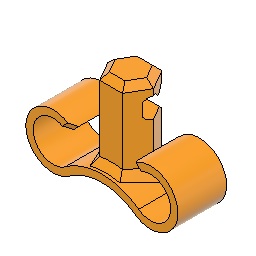
Prusament Clip v6 (Autodesk Fusion 360 design; units mm, degrees)
Autodesk Fusion 360 part; units mm, degrees
note: some values were not read from the file. Chosen so that the rebuilt part matches the saved one: which face or edge a step refers to; which pieces of a blend or face edit are solid. Set by a fixed rule: which sketch regions a step uses.
sketch "Sketch1" plane through (0, 0, 0) normal (0, 0, 1) x (1, 0, 0)
  line L0 (0, 0) -> (-8, 0)
  arc A0 (-5.3, 4.3077) -> (-8, 0) centre (-8, 3) ccw
  arc A1 (-4.22, 4.8307) -> (-8, -1.2) centre (-8, 3) ccw
  line L1 (0, -1.2) -> (-8, -1.2)
  line L2 (-5.3, 4.3077) -> (-4.22, 4.8307)
  line L3 (0, 2.5) -> (0, 20)
  arc A2 (8, 0) -> (5.3, 4.3077) centre (8, 3) ccw
  arc A3 (8, -1.2) -> (4.22, 4.8307) centre (8, 3) ccw
  line L4 (0, 0) -> (8, 0)
  line L5 (0, -1.2) -> (8, -1.2)
  line L6 (5.3, 4.3077) -> (4.22, 4.8307)
  dimension "d1" = 8
  dimension "d2" = 3
  dimension "d3" = 5.3
  dimension "d4" = 1.2
  constraint coincident L0.start L4.start
  constraint horizontal L0
  constraint tangent L0 A0
  constraint symmetric L0.start L3 L4.start
  constraint symmetric L0.end L3 A2.start
  constraint symmetric A0.start L3 A2.end
  constraint symmetric A0 L3 A2
  constraint symmetric A1.end L3 A3.start
  constraint symmetric A1.start L3 A3.end
  constraint symmetric A1 L3 A3
  constraint symmetric L1.start L3 L5.start
  measures "d1" distance of L0.start L0.end
  measures "d2" radius of A0
  measures "d3" horizontal distance of L0.start A0.start
extrude "Extrude1" add sketch "Sketch1" along normal blind 8 makes body 1
sketch "Sketch2" plane through (0, 0, 0) normal (0, 1, 0) x (-1, 0, 0)
  line L0 (-8, 0) -> (8, 0)
  line L1 (8, 0) -> (8, 8)
  line L2 (8, 8) -> (-8, 8)
  line L3 (-8, 8) -> (-8, 0)
  line L4 (1.875, 8) -> (-1.875, 8)
  line L5 (-1.875, 8) -> (-3.75, 4.7524)
  line L6 (-3.75, 4.7524) -> (-1.875, 1.5048)
  line L7 (-1.875, 1.5048) -> (1.875, 1.5048)
  line L8 (1.875, 1.5048) -> (3.75, 4.7524)
  line L9 (3.75, 4.7524) -> (1.875, 8)
  point P0 (0, 4.7524)
  dimension "d12" = 3.75
  constraint collinear L2 L4
  constraint vertical P0 origin
  measures "d12" distance of L4.start P0
extrude "Extrude2" add sketch "Sketch2" along normal blind 16 contours L2 L4 L5 L6 L7 L8 L9 bodies 1
sketch "Sketch5" plane through (0, 0, 1.5048) normal (0, 0, -1) x (-1, 0, 0)
  line L0 (-1.875, 0) -> (1.875, 0)
  line L1 (1.875, 0) -> (1.875, 16)
  line L2 (1.875, 16) -> (-1.875, 16)
  line L3 (-1.875, 16) -> (-1.875, 0)
  line L4 (-3.75, 11.97) -> (-1, 11.97)
  line L5 (-1, 11.97) -> (-1, 12.47)
  arc A0 (1, 12.47) -> (-1, 12.47) centre (0, 12.47) ccw
  line L6 (1, 12.47) -> (1, 9.97)
  line L7 (1, 9.97) -> (-3.75, 9.97)
  line L8 (-3.75, 9.97) -> (-3.75, 11.97)
  line L9 (0, 2.5) -> (0, 20)
  line L10 (-3.75, 0) -> (-3.75, 16) construction
  line L11 (3.75, 0) -> (3.75, 16) construction
  line L12 (0, 0) -> (-8, 0) construction
  point P0 (-3.75, 11.97)
  point P1 (0, 2.5)
  dimension "d27" = 2
  dimension "d29" = 1
  dimension "d30" = 11.97
  dimension "d31" = 0.5
  constraint perpendicular L3 L4
  constraint perpendicular L4 L5
  constraint tangent L5 A0
  constraint perpendicular L5 L7
  constraint parallel L6 L8
  constraint parallel L5 L6
  constraint tangent A0 L6
  constraint vertical A0.centre P1
  constraint coincident P0 L4.start
  constraint collinear L8 L10
  measures "d27" distance of P0 L7.end
  measures "d29" radius of A0
  measures "d30" distance of P0 L12
  measures "d31" distance of L4.end L5.end
extrude "Extrude4" cut sketch "Sketch5" against normal through all contours L3 L4 L7 L8 | L3 L4 L5 A0 L7 L9 | A0 L6 L7 L9 bodies 1
chamfer "Chamfer5" distance 1 angle 45 6 edges at (0, 16, 8) (2.8125, 16, 6.3762) (2.8125, 16, 3.1286) (0, 16, 1.5048) (-2.8125, 16, 3.1286) (-2.8125, 16, 6.3762) on bodies 1
chamfer "Chamfer6" distance 1 angle 45 4 edges at (2.8125, 11.97, 3.1286) (2.8125, 11.97, 6.3762) (2.8125, 9.97, 6.3762) (2.8125, 9.97, 3.1286) on bodies 1
chamfer "Chamfer2" distance 1 angle 45 4 edges at (4.76, 4.5692, 0) (4.76, 4.5692, 8) (-4.76, 4.5692, 8) (-4.76, 4.5692, 0) on bodies 1
fillet "Fillet1" radius 0.8 1 edges at (-1, 9.97, 4.7524) on bodies 1
fillet "Fillet2" radius 3 5 edges at (2.8125, 0, 6.3762) (2.8125, 0, 3.1286) (0, 0, 1.5048) (-2.8125, 0, 3.1286) (-2.8125, 0, 6.3762) on bodies 1
sketch "Sketch1 (2)" plane through (0, 0, 0) normal (0, 0, 1) x (1, 0, 0) in component "Prusa Clip 2"
  circle A0 centre (-8, 0) radius 4.5
  circle A1 centre (8, 0) radius 4.5
  line L0 (-8, 0) -> (8, 0) construction
  circle A2 centre (0, -10.8743) radius 9
  circle A3 centre (-8, 0) radius 3.3
  circle A4 centre (8, 0) radius 3.3
  circle A5 centre (0, -10.8743) radius 10.2
  line L1 (-8, 0) -> (-4.818, 3.182)
  line L2 (8, 0) -> (4.818, 3.182)
  dimension "d37" = 16
  dimension "d38" = 9
  dimension "d39" = 18
  dimension "d42" = 1.2
  dimension "d43" = 45
  dimension "d44" = 45
  constraint equal A0 A1
  constraint coincident A0.centre L0.start
  constraint coincident A1.centre L0.end
  constraint horizontal L0
  constraint midpoint origin L0
  constraint vertical origin A2.centre
  constraint tangent A0 A2
  constraint coincident A0 L1.end
  constraint coincident A1 L2.end
  measures "d37" distance of A0.centre A1.centre
  measures "d38" diameter of A0
  measures "d39" diameter of A2
  measures "d43" angle of L0 L1
  measures "d44" angle of L0 L2
extrude "Extrude1'" add sketch "Sketch1 (2)" along normal blind 8 separate body contours A0 A3 A5 L1 | A0 A1 A2 A5 | A0 A5 | A1 A5 | A1 A4 A5 L2 picked at (-8.3046, -4.0801) picked at (-3.028, -1.5769) picked at (5.3905, 3.149) makes body 2 in component "Prusa Clip 2"
sketch "Sketch2 (2)" plane through (0, 0, 0) normal (0, 1, 0) x (1, 0, 0) in component "Prusa Clip 2"
  line L0 (3.75, -3.2476) -> (1.875, 0)
  line L1 (1.875, 0) -> (-1.875, 0)
  line L2 (-1.875, 0) -> (-3.75, -3.2476)
  line L3 (-3.75, -3.2476) -> (-1.875, -6.4952)
  line L4 (-1.875, -6.4952) -> (1.875, -6.4952)
  line L5 (1.875, -6.4952) -> (3.75, -3.2476)
  line L6 (-6.0444, 0) -> (6.0444, 0)
  point P0 (0, -3.2476)
  dimension "d47" = 3.75
  constraint collinear L1 L6
  constraint vertical origin P0
  measures "d47" distance of L0.start P0
extrude "Extrude2'" add sketch "Sketch2 (2)" along normal blind 12 and the other way up to surface second end surface at (4.2606, -1.6067, 5.3333) on bodies 2 bodies 2 in component "Prusa Clip 2"
sketch "Sketch3" plane through (0, 0, 0) normal (1, 0, 0) x (0, 0, -1) in component "Prusa Clip 2"
  line L0 (0, -0.8481) -> (0, 12)
  line L1 (0, 12) -> (-3.2476, 12)
  line L2 (-3.2476, 12) -> (-3.2476, -1.3886)
  ellipse E0 centre (3.2476, -10.8743) end of major axis (-14.4193, -10.8743) minor radius 10.2 (0, -0.8481) -> (-3.2476, -1.3886) ccw construction
  line L3 (-3.2476, -1.3886) -> (-3.2476, 12)
  line L4 (-3.2476, 12) -> (-6.4952, 12)
  line L5 (-6.4952, 12) -> (-6.4952, -0.8481)
  ellipse E1 centre (-9.7428, -10.8743) end of major axis (7.9241, -10.8743) minor radius 10.2 (-3.2476, -1.3886) -> (-6.4952, -0.8481) ccw construction
  line L6 (0, 4.5) -> (0, -4.5)
  line L7 (0, 3.182) -> (-8, 3.182)
  line L8 (-8, 4.5) -> (-8, -4.5)
  line L9 (-8, -3.6248) -> (0, -3.6248)
  line L10 (0, 6.7) -> (-4.4476, 6.7)
  line L11 (-4.4476, 6.7) -> (-4.4476, 9.2)
  arc A0 (-2.0476, 9.2) -> (-4.4476, 9.2) centre (-3.2476, 9.2) ccw
  line L12 (-2.0476, 9.2) -> (-2.0476, 8.7)
  line L13 (-2.0476, 8.7) -> (0, 8.7)
  line L14 (0, 8.7) -> (0, 6.7)
  line L15 (-4.4476, 9.2) -> (-3.2476, 10.4)
  line L16 (-3.2476, 10.4) -> (-2.0476, 9.2)
  dimension "d52" = 1.2
  dimension "d53" = 2
  dimension "d54" = 0.5
  dimension "d55" = 4.7
  constraint perpendicular L2 L10
  constraint perpendicular L10 L11
  constraint tangent L11 A0
  constraint tangent A0 L12
  constraint perpendicular L10 L12
  constraint perpendicular L12 L13
  constraint parallel L11 L14
  constraint collinear L0 L14
  constraint vertical L1.end A0.centre
  constraint midpoint A0 L15.end
  measures "d52" radius of A0
  measures "d53" distance of L10.start L13.end
  measures "d54" distance of A0.start L12.end
  measures "d55" vertical distance of L8.start A0.centre
extrude "Extrude3" cut sketch "Sketch3" along normal through all and the other way through all contours L0 L2 L3 L10 L12 L13 L14 L16 | L2 L3 L10 L11 L15 bodies 2 in component "Prusa Clip 2"
chamfer "Chamfer1" distance 1 angle 45 6 edges at (-2.8125, 12, 4.8714) (-2.8125, 12, 1.6238) (2.8125, 12, 1.6238) (0, 12, 6.4952) (2.8125, 12, 4.8714) (0, 12, 0) on bodies 2 in component "Prusa Clip 2"
chamfer "Chamfer2'" distance 1 angle 45 2 edges at (0, 8.7, 0) (0, 6.7, 0) on bodies 2 in component "Prusa Clip 2"
chamfer "Chamfer3" distance 1 angle 45 4 edges at (5.2423, 2.7577, 0) (-5.2423, 2.7577, 0) (5.2423, 2.7577, 8) (-5.2423, 2.7577, 8) on bodies 2 in component "Prusa Clip 2"
chamfer "Chamfer4" distance 1 angle 45 5 edges at (2.8255, -1.0734, 1.6462) (2.8255, -1.0734, 4.849) (0, -0.6743, 6.4952) (-2.8255, -1.0734, 4.849) (-2.8255, -1.0734, 1.6462) on bodies 2 in component "Prusa Clip 2"
chamfer "Chamfer5'" distance 0.5 angle 45 1 edges at (0, 8.7, 2.0476) on bodies 2 in component "Prusa Clip 2"
chamfer "Chamfer6'" distance 0.5 angle 45 1 edges at (0, 6.7, 4.4476) on bodies 2 in component "Prusa Clip 2"
fillet "Fillet2'" radius 1 1 edges at (0, 10.4, 3.2476) on bodies 2 in component "Prusa Clip 2"
component "Prusa Clip 2" placed x (1, 0, 0) y (0, 1, 0) z (0, 0, 1) at (0, 0, 0)
equation "d2 = Rs"
equation "d4 = w"
equation "D = 7.5 mm" comment "Needle diameter."
equation "w = 1.2 mm" comment "Belt width"
equation "Rs = 3 mm" comment "Spring diameter"
equation "d12 = D / 2"
equation "d13 = 2 * Rs + w + 4.8 mm + 4 mm"
equation "d30 = 2 * Rs + w + 4.77 mm"
equation "d39 = d38 * 2"
equation "d40 = -w"
equation "d41 = -w"
equation "d42 = w"
equation "d44 = d43"
equation "d47 = D / 2"
named bodies: "Prusament Clip", "Prusament Clip Mk.2"
